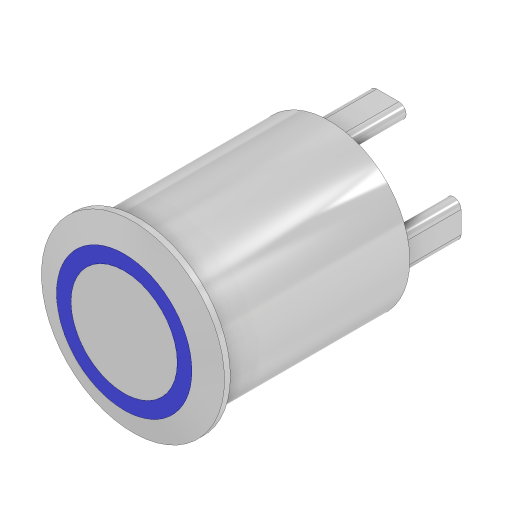
# Autodesk Inventor part: Кнопка
Saved by Autodesk Inventor 2023 (Build 270158000, 158)
## iProperties
Created: 2023-02-23
Part Number: Кнопка
Material: Типовые
Document SubType Name: Modeling
Designer: Admin
Density: 1 g/cm^3
Appearance: По умолчанию
Author: Admin
Autodesk Inventor part; units mm, degrees
ref_plane "YZ Plane" through (0, 0, 0) normal (1, 0, 0) x (0, 1, 0)
ref_plane "XZ Plane" through (0, 0, 0) normal (0, 1, 0) x (-1, 0, 0)
ref_plane "XY Plane" through (0, 0, 0) normal (0, 0, 1) x (1, 0, 0)
sketch "Эскиз1" plane through (0, 0, 0) normal (0, 0, 1) x (1, 0, 0)
  circle A0 centre (0, 0) radius 12.5
  circle A1 centre (0, 0) radius 9.25
  circle A2 centre (0, 0) radius 7.25
  dimension "d0" = 18.5
  dimension "d1" = 25
  dimension "d20" = 2
  constraints: 3 centre point, 3 coincident
  measures "d0" diameter of A1
  measures "d1" diameter of A0
  measures "d20" radial gap between concentric circles of A1 A2
extrude "Выдавливание1" add sketch "Эскиз1" against normal blind 2 contours A0 | A1 | A2
chamfer "Фаска1" distance 3.25 distance2 1.2 1 edges at (-12.5, 0, 0) measured on face at (-12, 0, 0)
sketch "Эскиз2" plane through (0, 0, -2) normal (0, 0, -1) x (-1, 0, 0)
  circle A0 centre (0, 0) radius 11
  dimension "d7" = 22
  constraints: 1 centre point, 1 coincident
  measures "d7" diameter of A0
extrude "Выдавливание2" add sketch "Эскиз2" along normal blind 26
sketch "Эскиз3" plane through (0, 0, -28) normal (0, 0, -1) x (-1, 0, 0)
  line L0 (-9, -1.5) -> (-9, 1.5) construction
  line L1 (-10, -1.5) -> (-10, 1.5)
  line L2 (-8, 1.5) -> (-8, -1.5)
  arc A0 (-10, -1.5) -> (-8, -1.5) centre (-9, -1.5) ccw
  arc A1 (-8, 1.5) -> (-10, 1.5) centre (-9, 1.5) ccw
  arc A2 (-1.5, -8) -> (-1.5, -10) centre (-1.5, -9) ccw
  line L3 (1.5, -10) -> (-1.5, -10)
  arc A3 (1.5, -10) -> (1.5, -8) centre (1.5, -9) ccw
  line L4 (-1.5, -8) -> (1.5, -8)
  arc A4 (8, -1.5) -> (10, -1.5) centre (9, -1.5) ccw
  line L5 (10, 1.5) -> (10, -1.5)
  arc A5 (10, 1.5) -> (8, 1.5) centre (9, 1.5) ccw
  line L6 (8, -1.5) -> (8, 1.5)
  arc A6 (1.5, 8) -> (1.5, 10) centre (1.5, 9) ccw
  line L7 (-1.5, 10) -> (1.5, 10)
  arc A7 (-1.5, 10) -> (-1.5, 8) centre (-1.5, 9) ccw
  line L8 (1.5, 8) -> (-1.5, 8)
  point P0 (0, 0)
  point P1 (-9, 0)
  dimension "d11" = 3
  dimension "d12" = 1
  dimension "d13" = 8
  dimension "d16" = 360
  constraints: 20 end point, 16 point on circle, 8 centre point, 4 tangent, 1 horizontal alignment, 1 midpoint, 1 parallel, 1 vertical, 41 other
  measures "d11" distance of L0.start L0.end
  measures "d12" radius of A1
  measures "d13" distance from line of point (0, 0) L2
extrude "Выдавливание3" add sketch "Эскиз3" along normal blind 8 separate body
extrude "Выдавливание4" cut sketch "Эскиз1" against normal blind 1 contours A1 bodies 1
extrude "Выдавливание5" add sketch "Эскиз1" against normal blind 1 separate body contours A1
